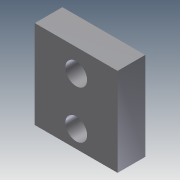
# Autodesk Inventor part: linacspacers
Saved by Autodesk Inventor 2011 (Build 150239000, 239)
## iProperties
Created: 2011-12-28
Part Number: linacspacers
Document SubType Name: Modeling
Designer: Matthew
Density: 1 g/cm^3
Author: Matthew
Autodesk Inventor part; units mm, degrees
ref_plane "YZ Plane" through (0, 0, 0) normal (1, 0, 0) x (0, 1, 0)
ref_plane "XZ Plane" through (0, 0, 0) normal (0, 1, 0) x (-1, 0, 0)
ref_plane "XY Plane" through (0, 0, 0) normal (0, 0, 1) x (1, 0, 0)
sketch "Sketch1" plane through (0, 0, 0) normal (0, 0, 1) x (1, 0, 0)
  line L0 (-16.3387, -16.9652) -> (21.7613, -16.9652)
  line L1 (21.7613, -16.9652) -> (21.7613, -57.6052)
  line L2 (21.7613, -57.6052) -> (-16.3387, -57.6052)
  line L3 (-16.3387, -57.6052) -> (-16.3387, -16.9652)
  point P0 (0, 0)
  dimension "d0" = 38.1
  dimension "d1" = 40.64
  constraints: 8 end point, 2 parallel, 1 horizontal, 1 perpendicular
  measures "d0" distance of L1.end L2.end
  measures "d1" distance of L0.end L1.end
extrude "Extrusion1" add sketch "Sketch1" along normal blind 12.7
sketch "Sketch2" plane through (0, 0, 12.7) normal (0, 0, 1) x (1, 0, 0)
  line L0 (21.7613, -57.6052) -> (-16.3387, -57.6052) projected
  line L1 (2.7113, -57.6052) -> (2.7113, -49.6052)
  circle A0 centre (2.7113, -49.6052) radius 5
  line L2 (2.7113, -57.6052) -> (2.7113, -27.6052)
  circle A1 centre (2.7113, -27.6052) radius 5
  point P0 (0, 0)
  dimension "d4" = 8
  dimension "d5" = 10
  dimension "d6" = 30
  constraints: 4 end point, 2 centre point, 2 coincident, 1 midpoint, 1 perpendicular, 1 point on line
  measures "d4" distance of L1.start L1.end
  measures "d5" diameter of A0
  measures "d6" distance of L1.start L2.end
extrude "Extrusion2" cut sketch "Sketch2" against normal blind 12.7
body "Solid1"
